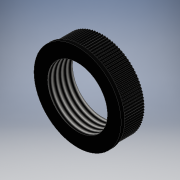
# Autodesk Inventor part: Toggle_Nut
Saved by Autodesk Inventor 2016 (Build 200138000, 138)
## iProperties
Created: 2016-04-13
Part Number: Toggle_Nut
Material: PC/ABS Plastic
Document SubType Name: Modeling
Designer: agmle
Density: 0.357273 g/cm^3
Appearance: Smooth - Black
Author: agmle
Autodesk Inventor part; units mm, degrees
ref_plane "YZ Plane" through (0, 0, 0) normal (1, 0, 0) x (0, 1, 0)
ref_plane "XZ Plane" through (0, 0, 0) normal (0, 1, 0) x (-1, 0, 0)
ref_plane "XY Plane" through (0, 0, 0) normal (0, 0, 1) x (1, 0, 0)
sketch "Sketch1" plane through (0, 0, 0) normal (0, 1, 0) x (-1, 0, 0)
  circle A0 centre (0, 0) radius 8.75
  circle A1 centre (0, 0) radius 6
  dimension "d0" = 17.5
  dimension "d1" = 12
  constraints: 2 centre point, 2 coincident
  measures "d0" diameter of A0
  measures "d1" diameter of A1
extrude "Extrusion1" add sketch "Sketch1" along normal blind 5
thread "Thread1" size "M12x1" class "6H" standard "ANSI Metric M Profile" full length
sketch "Sketch2" plane through (0, 5, 0) normal (0, 1, 0) x (1, 0, 0)
  circle A0 centre (0, 0) radius 8.25 construction
  circle A1 centre (0, 0) radius 8.45 construction
  line L0 (-8.45, 0) -> (-8.2462, -0.25)
  line L1 (-8.45, 0) -> (-8.2462, 0.25)
  line L2 (-8.45, 0) -> (0, 0) construction
  line L3 (-8.2462, -0.25) -> (0, 0) construction
  line L4 (-8.2462, 0.25) -> (0, 0) construction
  line L5 (-8.2462, -0.25) -> (-8.746, -0.2652)
  circle A2 centre (0, 0) radius 8.75 projected
  line L6 (-8.2462, 0.25) -> (-8.746, 0.2652)
  dimension "d6" = 16.9
  dimension "d7" = 16.5
  dimension "d8" = 0.5
  constraints: 14 end point, 4 point on circle, 2 coincident, 2 collinear, 1 centre point, 1 equal length, 1 horizontal, 1 horizontal alignment, 2 other
  measures "d7" diameter of A0
  measures "d8" distance of L1.end L0.end
extrude "Extrusion2" cut sketch "Sketch2" against normal blind 4.3 contours L0 L5 A2 L6 L1 picked at (-8.4807, -0.1717)
pattern_circular "Circular Pattern1" count 104 over 360 about axis through (0, 0, 0) along (0, 1, 0) of "Extrusion2"
body "Solid1"
